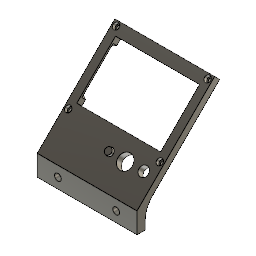
lcd-bracket (Autodesk Fusion 360 design; units mm, degrees)
Autodesk Fusion 360 part; units mm, degrees
note: some values were not read from the file. Chosen so that the rebuilt part matches the saved one: a direction. Set by a fixed rule: which sketch regions a step uses.
sketch "usable" plane through (0, 0, 0) normal (0, 0, 1) x (1, 0, 0) in component "lcd"
  line L0 (92.082, 84.258) -> (91.891, 83.734)
  line L1 (2.5, 82.931) -> (1.9507, 83.028)
  line L2 (3.5324, 85.767) -> (3.891, 85.34)
  line L3 (4.0817, 84.816) -> (4.0817, 84.258)
  line L4 (3.891, 85.34) -> (4.0817, 84.816)
  line L5 (1.4676, 83.307) -> (1.1091, 83.734)
  line L6 (3.891, 83.734) -> (3.5324, 83.307)
  line L7 (4.0817, 84.258) -> (3.891, 83.734)
  line L8 (91.532, 85.767) -> (91.891, 85.34)
  line L9 (91.891, 85.34) -> (92.082, 84.816)
  line L10 (0, 0) -> (93, 0)
  line L11 (89.109, 85.34) -> (89.468, 85.767)
  line L12 (3.0493, 86.046) -> (3.5324, 85.767)
  line L13 (1.9507, 86.046) -> (2.5, 86.143)
  line L14 (2.5, 86.143) -> (3.0493, 86.046)
  line L15 (89.109, 83.734) -> (88.918, 84.258)
  line L16 (3.5324, 83.307) -> (3.0493, 83.028)
  line L17 (89.951, 83.028) -> (89.468, 83.307)
  line L18 (91.049, 86.046) -> (91.532, 85.767)
  line L19 (91.891, 83.734) -> (91.532, 83.307)
  line L20 (90.5, 82.931) -> (89.951, 83.028)
  line L21 (90.5, 86.143) -> (91.049, 86.046)
  line L22 (91.532, 83.307) -> (91.049, 83.028)
  line L23 (93, 0) -> (93, 87)
  line L24 (0, 0) -> (0, 87)
  line L25 (91.049, 83.028) -> (90.5, 82.931)
  line L26 (1.4676, 85.767) -> (1.9507, 86.046)
  line L27 (89.468, 83.307) -> (89.109, 83.734)
  line L28 (0, 87) -> (93, 87)
  line L29 (88.918, 84.258) -> (88.918, 84.816)
  line L30 (89.951, 86.046) -> (90.5, 86.143)
  line L31 (92.082, 84.816) -> (92.082, 84.258)
  line L32 (89.468, 85.767) -> (89.951, 86.046)
  line L33 (88.918, 84.816) -> (89.109, 85.34)
  line L34 (1.9507, 83.028) -> (1.4676, 83.307)
  line L35 (3.0493, 83.028) -> (2.5, 82.931)
  line L36 (0.9183, 84.258) -> (0.9183, 84.816)
  line L37 (0.9183, 84.816) -> (1.1091, 85.34)
  line L38 (1.1091, 85.34) -> (1.4676, 85.767)
  line L39 (1.1091, 83.734) -> (0.9183, 84.258)
  line L40 (91.532, 20.7674) -> (91.891, 20.3401)
  line L41 (91.049, 21.0463) -> (91.532, 20.7674)
  line L42 (1.1091, 18.734) -> (0.9183, 19.2581)
  line L43 (1.1091, 20.3401) -> (1.4676, 20.7674)
  line L44 (3.5324, 20.7674) -> (3.891, 20.3401)
  line L45 (89.951, 21.0463) -> (90.5, 21.1431)
  line L46 (91.532, 18.3067) -> (91.049, 18.0278)
  line L47 (3.891, 18.734) -> (3.5324, 18.3067)
  line L48 (1.4676, 20.7674) -> (1.9507, 21.0463)
  line L49 (88.918, 19.8159) -> (89.109, 20.3401)
  line L50 (4.0817, 19.8159) -> (4.0817, 19.2581)
  line L51 (91.891, 20.3401) -> (92.082, 19.8159)
  line L52 (1.4676, 18.3067) -> (1.1091, 18.734)
  line L53 (2.5, 17.9309) -> (1.9507, 18.0278)
  line L54 (3.5324, 18.3067) -> (3.0493, 18.0278)
  line L55 (91.891, 18.734) -> (91.532, 18.3067)
  line L56 (92.082, 19.2581) -> (91.891, 18.734)
  line L57 (89.468, 18.3067) -> (89.109, 18.734)
  line L58 (89.109, 20.3401) -> (89.468, 20.7674)
  line L59 (0.9183, 19.2581) -> (0.9183, 19.8159)
  line L60 (90.5, 21.1431) -> (91.049, 21.0463)
  line L61 (92.082, 19.8159) -> (92.082, 19.2581)
  line L62 (88.918, 19.2581) -> (88.918, 19.8159)
  line L63 (90.5, 17.9309) -> (89.951, 18.0278)
  line L64 (3.0493, 18.0278) -> (2.5, 17.9309)
  line L65 (0.9183, 19.8159) -> (1.1091, 20.3401)
  line L66 (4.0817, 19.2581) -> (3.891, 18.734)
  line L67 (89.951, 18.0278) -> (89.468, 18.3067)
  line L68 (3.891, 20.3401) -> (4.0817, 19.8159)
  line L69 (89.468, 20.7674) -> (89.951, 21.0463)
  line L70 (91.049, 18.0278) -> (90.5, 17.9309)
  line L71 (1.9507, 18.0278) -> (1.4676, 18.3067)
  line L72 (89.109, 18.734) -> (88.918, 19.2581)
  line L73 (3.0493, 21.0463) -> (3.5324, 20.7674)
  line L74 (2.5, 21.1431) -> (3.0493, 21.0463)
  line L75 (1.9507, 21.0463) -> (2.5, 21.1431)
sketch "Sketch2" plane through (0, 0, 0) normal (0, 0, 1) x (1, 0, 0) in component "lcd"
  circle A0 centre (90.4999, 84.5371) radius 1.6
  circle A1 centre (2.4998, 84.537) radius 1.6
  line L0 (0, 0) -> (0, 87)
  line L1 (0, 87) -> (93, 87)
  line L2 (93, 0) -> (93, 87)
  line L3 (0, 0) -> (93, 0)
  line L4 (88.8, 14.5) -> (88.8, 2.5)
  line L5 (88.8, 2.5) -> (76.8, 2.5)
  line L6 (76.8, 2.5) -> (76.8, 14.5)
  line L7 (76.8, 14.5) -> (88.8, 14.5)
  circle A2 centre (82.8, 8.5) radius 3.5
  line L8 (88.8, 8.5) -> (76.8, 8.5) construction
  line L9 (82.8, 14.5) -> (82.8, 2.5) construction
  circle A3 centre (65.45, 7.85) radius 5.85
  line L10 (47.1, 11.55) -> (53.35, 11.55)
  line L11 (53.35, 11.55) -> (53.35, 5.3)
  line L12 (53.35, 5.3) -> (47.1, 5.3)
  line L13 (47.1, 5.3) -> (47.1, 11.55)
  circle A4 centre (2.5, 19.537) radius 1.6
  circle A5 centre (90.4998, 19.537) radius 1.6
  dimension "d24" = 4.2
  dimension "d25" = 2.5
  dimension "d26" = 12
  dimension "d27" = 12
  dimension "d28" = 7
  dimension "d29" = 11.7
  dimension "d30" = 2
  dimension "d31" = 5.5
  dimension "d32" = 5.3
  dimension "d33" = 6.25
  dimension "d34" = 6.25
  dimension "d35" = 47.1
  dimension "d71" = 3.2
  dimension "d72" = 3.2
  dimension "d73" = 3.2
  dimension "d74" = 3.2
  measures "d24" distance of L2 L4
  measures "d25" distance of L3 L5
  measures "d26" distance of L4 L6
  measures "d27" distance of L5 L7
  measures "d28" diameter of A2
  measures "d29" diameter of A3
  measures "d32" distance of L3 L12
  measures "d33" distance of L11 L13
  measures "d34" distance of L10 L12
  measures "d35" distance of L0 L13
  measures "d71" diameter of A0
  measures "d72" diameter of A1
  measures "d73" diameter of A4
  measures "d74" diameter of A5
extrude "Extrude1" add sketch "Sketch2" along normal blind 1.65 contours L0 L1 L2 L3 | L4 L5 L6 L7 | A2 | A3 | L10 L11 L12 L13 makes body 1 in component "lcd"
ref_plane "WorkPlane1" through (46.5, 43.5, 8.35) normal (0, 0, 1) x (1, 0, 0) in component "lcd"
sketch "Sketch3" plane through (46.5, 43.5, 8.35) normal (0, 0, 1) x (1, 0, 0) in component "lcd"
  line L0 (-46.5, -43.5) -> (46.5, -43.5)
  line L1 (-46.5, 43.5) -> (-46.5, -43.5)
  line L2 (46.5, -43.5) -> (46.5, 43.5)
  line L3 (46.5, 43.5) -> (-46.5, 43.5)
  line L4 (-46.5, -26.3) -> (46.5, -26.3)
  line L5 (39.3, 33.9) -> (39.3, -16.7)
  line L6 (39.3, -16.7) -> (-39.2, -16.7)
  line L7 (39.3, 33.9) -> (-39.2, 33.9)
  line L8 (-45.9, 25.1) -> (-45.9, -7.9)
  line L9 (-45.9, -7.9) -> (-39.2, -11.7)
  line L10 (-39.2, -11.7) -> (-39.2, -16.7)
  line L11 (-45.9, 25.1) -> (-39.2, 28.9)
  line L12 (-39.2, 28.9) -> (-39.2, 33.9)
  line L13 (-39.2, 28.9) -> (-39.2, -11.7)
  circle A0 centre (-44.0002, 41.037) radius 1.6
  circle A1 centre (43.9999, 41.0371) radius 1.6
  circle A2 centre (43.9998, -23.963) radius 1.6
  circle A3 centre (-44, -23.963) radius 1.6
  dimension "d5" = 17.2
  dimension "d6" = 7.2
  dimension "d7" = 9.6
  dimension "d8" = 9.6
  dimension "d10" = 7.3
  dimension "d11" = 33
  dimension "d12" = 6.7
  dimension "d13" = 5
  measures "d5" distance of L0 L4
  measures "d6" distance of L2 L5
  measures "d7" distance of L4 L6
  measures "d8" distance of L3 L7
  measures "d11" distance of origin
  measures "d12" distance of L8 L10
extrude "Extrude3" add sketch "Sketch3" along normal blind 1.6 separate body contours L1 L2 L3 L4 | L5 L6 L7 L10 L12 L13 | L8 L9 L11 L13 makes body 2 in component "lcd"
extrude "Extrude4" add sketch "Sketch3" along normal blind 3.7 from surface at 1.6 contours L8 L9 L11 L13 bodies 2 in component "lcd"
extrude "Extrude5" add sketch "Sketch3" along normal blind 8.6 from surface at 1.6 contours L5 L6 L7 L10 L12 L13 bodies 2 in component "lcd"
extrude "Extrude6" add sketch "Sketch2" along normal blind 4 from surface at 1.65 contours L10 L11 L12 L13 bodies 1 in component "lcd"
extrude "Extrude7" add sketch "Sketch2" along normal blind 9.5 from surface at 1.65 contours A3 bodies 1 in component "lcd"
extrude "Extrude8" add sketch "Sketch2" along normal blind 5.2 from surface at 1.65 contours L4 L5 L6 L7 bodies 1 in component "lcd"
extrude "Extrude9" add sketch "Sketch2" along normal blind 24.3 from surface at 1.65 contours A2 bodies 1 in component "lcd"
sketch "Sketch1" plane through (0, 0, 9.95) normal (0, 0, 1) x (-1, 0, 0) in component "bracket"
  line L0 (1.5, -88.5) -> (-94.5, -88.5)
  line L1 (-94.5, -88.5) -> (-94.5, 1.5)
  line L2 (-94.5, 1.5) -> (1.5, 1.5)
  line L3 (1.5, 1.5) -> (1.5, -88.5)
  line L4 (0, -87) -> (0, 0) construction
  line L5 (0, 0) -> (-93, 0) construction
  line L6 (-93, 0) -> (-93, -87) construction
  line L7 (-93, -87) -> (0, -87) construction
  circle A0 centre (-90.4999, -84.5371) radius 1.6
  circle A1 centre (-2.4998, -84.537) radius 1.6
  line L8 (-47.1, -11.55) -> (-53.35, -11.55) construction
  line L9 (-53.35, -11.55) -> (-53.35, -5.3) construction
  line L10 (-53.35, -5.3) -> (-47.1, -5.3) construction
  line L11 (-47.1, -5.3) -> (-47.1, -11.55) construction
  circle A2 centre (-65.45, -7.85) radius 5.85 construction
  line L12 (-88.8, -14.5) -> (-88.8, -2.5) construction
  line L13 (-88.8, -2.5) -> (-76.8, -2.5) construction
  line L14 (-76.8, -2.5) -> (-76.8, -14.5) construction
  line L15 (-76.8, -14.5) -> (-88.8, -14.5) construction
  line L16 (0, -87) -> (-93, 0) construction
  line L17 (0, 0) -> (-93, -87) construction
  line L18 (1.5, 1.5) -> (-94.5, -88.5) construction
  line L19 (-94.5, 1.5) -> (1.5, -88.5) construction
  circle A3 centre (-82.8, -8.5) radius 3.5 construction
  circle A4 centre (-82.8, -8.5) radius 4.5
  circle A5 centre (-65.45, -7.85) radius 6.85
  circle A6 centre (-2.5, -19.537) radius 2.9
  circle A7 centre (-90.4998, -19.537) radius 2.9
  circle A8 centre (-90.4999, -84.5371) radius 2.9
  circle A9 centre (-2.4998, -84.537) radius 2.9
  line L20 (-0.6, -35.6) -> (-7.3, -31.8)
  line L21 (-0.6, -68.6) -> (-0.6, -35.6)
  line L22 (-7.3, -72.4) -> (-0.6, -68.6)
  line L23 (-85.8, -26.8) -> (-85.8, -77.4)
  line L24 (-85.8, -77.4) -> (-7.3, -77.4)
  line L25 (-7.3, -77.4) -> (-7.3, -26.8)
  line L26 (-7.3, -26.8) -> (-85.8, -26.8)
  line L27 (-86.8, -78.4) -> (-6.3, -78.4)
  line L28 (-6.3, -78.4) -> (-6.3, -25.8)
  line L29 (-6.3, -25.8) -> (-86.8, -25.8)
  line L30 (-86.8, -25.8) -> (-86.8, -78.4)
  line L31 (-6.6833, -73.4873) -> (0.65, -69.3281)
  line L32 (0.65, -69.3281) -> (0.65, -34.8719)
  line L33 (0.65, -34.8719) -> (-6.6833, -30.7127)
  line L34 (-53.35, -5.3) -> (-47.1, -11.55) construction
  line L35 (-47.1, -5.3) -> (-53.35, -11.55) construction
  circle A10 centre (-50.225, -8.425) radius 4.5
  circle A11 centre (-50.225, -8.425) radius 3.5
  line L36 (-6.6833, -30.7127) -> (-7.3, -30.3629)
  line L37 (-6.6833, -73.4873) -> (-7.3, -73.8371)
  circle A12 centre (-90.4998, -19.537) radius 1.6
  circle A13 centre (-2.5, -19.537) radius 1.6
  dimension "d48" = 96
  dimension "d49" = 90
  dimension "d50" = 1
  dimension "d51" = 1
  dimension "d52" = 5.8
  dimension "d53" = 5.8
  dimension "d54" = 5.8
  dimension "d55" = 5.8
  dimension "d56" = 1
  dimension "d57" = 1.25
  dimension "d60" = 9
  dimension "d61" = 7
  measures "d48" distance of L1 L3
  measures "d49" distance of L0 L2
  measures "d50" distance of A3 A4
  measures "d51" distance of A2 A5
  measures "d52" diameter of A6
  measures "d53" diameter of A7
  measures "d54" diameter of A9
  measures "d55" diameter of A8
  measures "d56" distance of L24
  measures "d57" distance of L22
  measures "d60" diameter of A10
  measures "d61" diameter of A11
extrude "Extrude1'" add sketch "Sketch1" along normal blind 7 separate body contours L0 L1 L2 L3 | A6 | A7 | A8 | A9 | A10 makes body 3 in component "bracket"
extrude "Extrude2" cut sketch "Sketch1" against normal blind 3.7 from surface at 7 contours A6 | A7 | A8 | A9 | A12 | A13 bodies 3 in component "bracket"
extrude "Extrude4'" add sketch "Sketch1" along normal up to surface (2 mm away) from surface at 5 contours L20 L21 L22 L28 | L20 L21 L22 L28 L31 L32 L33 bodies 3 in component "bracket"
sketch "Sketch2 (2)" plane through (0, 0, 0) normal (1, 0, 0) x (0, 0.707107, -0.707107) in component "bracket"
  line L0 (55.5432, 69.6147) -> (-8.0964, 5.9751)
  line L1 (-24.0964, -0.1255) -> (-13.0461, 10.9248)
  line L2 (-13.0461, 10.9248) -> (-8.0964, 5.9751)
  line L3 (-13.0461, 10.9248) -> (50.5935, 74.5644)
  line L4 (-16.0964, -20.1255) -> (-24.0964, -20.1255)
  line L5 (-24.0964, -20.1255) -> (-24.0964, -0.1255)
  arc A0 (-8.774, 5.2974) -> (-16.0964, -12.3803) centre (8.9036, -12.3803) ccw
  line L6 (-8.0964, 5.9751) -> (-16.0964, -2.0249)
  line L7 (-16.0964, -2.0249) -> (-16.0964, -20.1255)
  dimension "d89" = 25
  dimension "d91" = 20
  dimension "d100" = 8
  dimension "d101" = 16
  measures "d89" radius of A0
  measures "d91" distance of L4 origin
  measures "d100" distance of origin
  measures "d101" distance of origin
extrude "Extrude5'" add sketch "Sketch2 (2)" along normal up to surface (94.5 mm away) and the other way up to surface (1.5 mm away) bodies 3 in component "bracket"
sketch "Sketch1 (2)" plane through (0, -11.3819, 11.3819) normal (0, 0.707107, -0.707107) x (-1, 0, 0) in component "bracket"
  circle A0 centre (-74.5, -10.1255) radius 3.25
  circle A1 centre (-18.5, -10.1255) radius 3.25
  line L0 (-74.5, -20.1255) -> (-74.5, -0.1255) construction
  line L1 (-18.5, -20.1255) -> (-18.5, -0.1255) construction
  line L2 (-74.5, -10.1255) -> (-94.5, -10.1255) construction
  line L3 (-18.5, -10.1255) -> (1.5, -10.1255) construction
  circle A2 centre (-74.5, -10.1255) radius 4.6
  circle A3 centre (-18.5, -10.1255) radius 4.6
  line L4 (-94.5, -20.1255) -> (-94.5, -0.1255) construction
  line L5 (1.5, -0.1255) -> (1.5, -20.1255) construction
  line L6 (1.5, -0.1255) -> (-94.5, -0.1255) construction
  line L7 (1.5, -20.1255) -> (-94.5, -20.1255) construction
  dimension "d92" = 6.5
  dimension "d93" = 6.5
  dimension "d95" = 9.2
  dimension "d96" = 9.2
  dimension "d102" = 20
  measures "d92" diameter of A0
  measures "d93" diameter of A1
  measures "d95" diameter of A2
  measures "d96" diameter of A3
extrude "Extrude8'" cut sketch "Sketch1 (2)" along normal through all contours A0 | A1 | A2 | A3 bodies 3 in component "bracket"
extrude "Extrude9'" cut sketch "Sketch1 (2)" against normal through all contours A0 | A1 bodies 3 in component "bracket"
ref_plane "WorkPlane1" through (46.5, 43.0208, 7.95) normal (0, 0, -1) x (1, 0, 0) in component "bracket"
sketch "Sketch4" plane through (50.225, 8.425, 7.95) normal (0, 0, -1) x (1, 0, 0) in component "bracket"
  circle A0 centre (0, 0) radius 3.1
  circle A1 centre (0, 0) radius 4.1
  circle A2 centre (0, 0) radius 3.5 construction
  dimension "d111" = 0.4
  dimension "d112" = 0.6
  measures "d111" distance of A0 A2
  measures "d112" distance of A1 A2
extrude "Extrude10" add sketch "Sketch4" against normal up to surface (11 mm away) separate body contours A0 makes body 4 in component "bracket"
extrude "Extrude11" add sketch "Sketch4" against normal up to surface (2 mm away) contours A0 | A1 bodies 4 in component "bracket"
component "lcd" placed x (1, 0, 0) y (0, 0.707107, 0.707107) z (0, -0.707107, 0.707107) at (0, 0, 0)
component "bracket" placed x (1, 0, 0) y (0, 0.707107, 0.707107) z (0, -0.707107, 0.707107) at (0, 0, 0)
equation "d8 = d7"
equation "d34 = d33"
equation "d53 = d52"
equation "d54 = d52"
equation "d55 = d52"
equation "d72 = d71"
equation "d73 = d71"
equation "d74 = d71"
named bodies: "main", "button"
